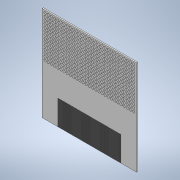
# Autodesk Inventor part: CeramicPCB_Coarse
Saved by Autodesk Inventor 2021 (Build 250183000, 183)
## iProperties
Created: 2021-11-05
Part Number: CeramicPCB_Coarse
Material: Generic
Document SubType Name: Sheet Metal
Designer: Unit-005
Density: 1 g/cm^3
Sheet Metal Rule: Default
Appearance: Default
Author: Unit-005
Autodesk Inventor part; units mm, degrees
ref_plane "YZ Plane" through (0, 0, 0) normal (1, 0, 0) x (0, 1, 0)
ref_plane "XZ Plane" through (0, 0, 0) normal (0, 1, 0) x (-1, 0, 0)
ref_plane "XY Plane" through (0, 0, 0) normal (0, 0, 1) x (1, 0, 0)
sketch "Sketch1" plane through (0, 0, 0) normal (0, 0, 1) x (1, 0, 0)
  line L0 (-38, 38) -> (38, 38)
  line L1 (38, 38) -> (38, -38)
  line L2 (38, -38) -> (-38, -38)
  line L3 (-38, -38) -> (-38, 38)
  line L4 (-38, 38) -> (38, -38) construction
  line L5 (38, 38) -> (-38, -38) construction
  point P0 (0, 0)
  dimension "d0" = 76
  dimension "d1" = 76
  constraints: 12 end point, 2 midpoint, 2 parallel, 1 horizontal, 1 perpendicular
  measures "d0" distance of L1.end L2.end
  measures "d1" distance of L0.end L1.end
extrude "Extrusion1" add sketch "Sketch1" along normal blind 1
sketch "Sketch2" plane through (0, 0, 1) normal (0, 0, 1) x (1, 0, 0)
  line L0 (-38, -38) -> (38, -38) projected
  line L1 (38, -38) -> (38, 38) projected
  line L2 (38, 38) -> (-38, 38) projected
  line L3 (-38, 38) -> (-38, -38) projected
  line L4 (-53.2, 0) -> (53.2, 0) projected
  line L5 (0, -53.2) -> (0, 53.2) projected
  line L6 (-0.15, -18) -> (0.15, -18)
  line L7 (0.15, -18) -> (0.15, -38)
  line L8 (0.15, -38) -> (-0.15, -38)
  line L9 (-0.15, -38) -> (-0.15, -18)
  line L10 (-0.15, -18) -> (0.15, -38) construction
  line L11 (0.15, -18) -> (-0.15, -38) construction
  line L12 (-38, -38) -> (38, -38) projected
  point P0 (0, 0)
  point P1 (0, -28)
  dimension "d4" = 0.3
  dimension "d5" = 20
  constraints: 12 end point, 2 midpoint, 2 parallel, 1 collinear, 1 horizontal, 1 perpendicular, 1 point on line
  measures "d4" distance of L7.end L8.end
  measures "d5" distance of L6.end L7.end
extrude "Extrusion2" add sketch "Sketch2" along normal blind 0.035 contours L9 L6 L5 L0 | L5 L6 L7 L0
pattern_linear "Rectangular Pattern1" count 85 spacing 0.6 along (1, 0, 0) of "Extrusion2" first direction both ways yes
sketch "Sketch3" plane through (0, 0, 1) normal (0, 0, 1) x (1, 0, 0)
  line L0 (0.15, -38) -> (0.45, -38) projected
  line L1 (38, -38) -> (38, 38) projected
  line L2 (38, 38) -> (-38, 38) projected
  line L3 (-38, 38) -> (-38, -38) projected
  line L4 (-38, -38) -> (-25.35, -38) projected
  line L5 (-53.2, 0) -> (53.2, 0) projected
  line L6 (0, -53.2) -> (0, 53.2) projected
  line L7 (33, -38) -> (33, 2) construction
  line L8 (-25.05, -38) -> (-24.75, -38) projected
  line L9 (-24.45, -38) -> (-24.15, -38) projected
  line L10 (-22.35, -38) -> (-22.35, -18) projected
  line L11 (-22.35, -18) -> (-22.05, -18) projected
  line L12 (-22.05, -18) -> (-22.05, -38) projected
  line L13 (-22.05, -38) -> (-21.75, -38) projected
  line L14 (-21.75, -38) -> (-21.75, -18) projected
  line L15 (-21.75, -18) -> (-21.45, -18) projected
  line L16 (-21.45, -18) -> (-21.45, -38) projected
  line L17 (-21.45, -38) -> (-21.15, -38) projected
  line L18 (-21.15, -38) -> (-21.15, -18) projected
  line L19 (-21.15, -18) -> (-20.85, -18) projected
  line L20 (-20.85, -18) -> (-20.85, -38) projected
  line L21 (-20.85, -38) -> (-20.55, -38) projected
  line L22 (-20.55, -38) -> (-20.55, -18) projected
  line L23 (-20.55, -18) -> (-20.25, -18) projected
  line L24 (-20.25, -18) -> (-20.25, -38) projected
  line L25 (-20.25, -38) -> (-19.95, -38) projected
  line L26 (-19.95, -38) -> (-19.95, -18) projected
  line L27 (-19.95, -18) -> (-19.65, -18) projected
  line L28 (-19.65, -18) -> (-19.65, -38) projected
  line L29 (-19.65, -38) -> (-19.35, -38) projected
  line L30 (-19.35, -38) -> (-19.35, -18) projected
  line L31 (-19.35, -18) -> (-19.05, -18) projected
  line L32 (-19.05, -18) -> (-19.05, -38) projected
  line L33 (-19.05, -38) -> (-18.75, -38) projected
  line L34 (-18.75, -38) -> (-18.75, -18) projected
  line L35 (-18.75, -18) -> (-18.45, -18) projected
  line L36 (-18.45, -18) -> (-18.45, -38) projected
  line L37 (-18.45, -38) -> (-18.15, -38) projected
  line L38 (-18.15, -38) -> (-18.15, -18) projected
  line L39 (-18.15, -18) -> (-17.85, -18) projected
  line L40 (-17.85, -18) -> (-17.85, -38) projected
  line L41 (-17.85, -38) -> (-17.55, -38) projected
  line L42 (-17.55, -38) -> (-17.55, -18) projected
  line L43 (-17.55, -18) -> (-17.25, -18) projected
  line L44 (-17.25, -18) -> (-17.25, -38) projected
  line L45 (-17.25, -38) -> (-16.95, -38) projected
  line L46 (-16.95, -38) -> (-16.95, -18) projected
  line L47 (-16.95, -18) -> (-16.65, -18) projected
  line L48 (-16.65, -18) -> (-16.65, -38) projected
  line L49 (-16.65, -38) -> (-16.35, -38) projected
  line L50 (-16.35, -38) -> (-16.35, -18) projected
  line L51 (-16.35, -18) -> (-16.05, -18) projected
  line L52 (-16.05, -18) -> (-16.05, -38) projected
  line L53 (-16.05, -38) -> (-15.75, -38) projected
  line L54 (-15.75, -38) -> (-15.75, -18) projected
  line L55 (-15.75, -18) -> (-15.45, -18) projected
  line L56 (-15.45, -18) -> (-15.45, -38) projected
  line L57 (-15.15, -38) -> (-15.15, -18) projected
  line L58 (-15.15, -18) -> (-14.85, -18) projected
  line L59 (-14.85, -18) -> (-14.85, -38) projected
  line L60 (-14.85, -38) -> (-14.55, -38) projected
  line L61 (-14.55, -38) -> (-14.55, -18) projected
  line L62 (-14.55, -18) -> (-14.25, -18) projected
  line L63 (-14.25, -18) -> (-14.25, -38) projected
  line L64 (-14.25, -38) -> (-13.95, -38) projected
  line L65 (-13.95, -38) -> (-13.95, -18) projected
  line L66 (-13.95, -18) -> (-13.65, -18) projected
  line L67 (-13.65, -18) -> (-13.65, -38) projected
  line L68 (-13.65, -38) -> (-13.35, -38) projected
  line L69 (-13.35, -38) -> (-13.35, -18) projected
  line L70 (-13.35, -18) -> (-13.05, -18) projected
  line L71 (-13.05, -18) -> (-13.05, -38) projected
  line L72 (-13.05, -38) -> (-12.75, -38) projected
  line L73 (-12.75, -38) -> (-12.75, -18) projected
  line L74 (-12.75, -18) -> (-12.45, -18) projected
  line L75 (-12.45, -18) -> (-12.45, -38) projected
  line L76 (-12.45, -38) -> (-12.15, -38) projected
  line L77 (-12.15, -38) -> (-12.15, -18) projected
  line L78 (-12.15, -18) -> (-11.85, -18) projected
  line L79 (-11.85, -18) -> (-11.85, -38) projected
  line L80 (-11.85, -38) -> (-11.55, -38) projected
  line L81 (-11.55, -38) -> (-11.55, -18) projected
  line L82 (-11.55, -18) -> (-11.25, -18) projected
  line L83 (-11.25, -18) -> (-11.25, -38) projected
  line L84 (-11.25, -38) -> (-10.95, -38) projected
  line L85 (-10.95, -38) -> (-10.95, -18) projected
  line L86 (-10.95, -18) -> (-10.65, -18) projected
  line L87 (-10.65, -18) -> (-10.65, -38) projected
  line L88 (-10.65, -38) -> (-10.35, -38) projected
  line L89 (-10.35, -38) -> (-10.35, -18) projected
  line L90 (-10.35, -18) -> (-10.05, -18) projected
  line L91 (-10.05, -18) -> (-10.05, -38) projected
  line L92 (-10.05, -38) -> (-9.75, -38) projected
  line L93 (-9.75, -38) -> (-9.75, -18) projected
  line L94 (-9.75, -18) -> (-9.45, -18) projected
  line L95 (-9.45, -18) -> (-9.45, -38) projected
  line L96 (-9.45, -38) -> (-9.15, -38) projected
  line L97 (-9.15, -38) -> (-9.15, -18) projected
  line L98 (-9.15, -18) -> (-8.85, -18) projected
  line L99 (-8.85, -18) -> (-8.85, -38) projected
  line L100 (-8.85, -38) -> (-8.55, -38) projected
  line L101 (-8.55, -38) -> (-8.55, -18) projected
  line L102 (-8.55, -18) -> (-8.25, -18) projected
  line L103 (-8.25, -18) -> (-8.25, -38) projected
  line L104 (-8.25, -38) -> (-7.95, -38) projected
  line L105 (-7.95, -38) -> (-7.95, -18) projected
  line L106 (-7.95, -18) -> (-7.65, -18) projected
  line L107 (-7.65, -18) -> (-7.65, -38) projected
  line L108 (-7.65, -38) -> (-7.35, -38) projected
  line L109 (-7.35, -38) -> (-7.35, -18) projected
  line L110 (-7.35, -18) -> (-7.05, -18) projected
  line L111 (-7.05, -18) -> (-7.05, -38) projected
  line L112 (-7.05, -38) -> (-6.75, -38) projected
  line L113 (-6.75, -38) -> (-6.75, -18) projected
  line L114 (-6.75, -18) -> (-6.45, -18) projected
  line L115 (-6.45, -18) -> (-6.45, -38) projected
  line L116 (-6.45, -38) -> (-6.15, -38) projected
  line L117 (-6.15, -38) -> (-6.15, -18) projected
  line L118 (-6.15, -18) -> (-5.85, -18) projected
  line L119 (-5.85, -18) -> (-5.85, -38) projected
  line L120 (-5.85, -38) -> (-5.55, -38) projected
  line L121 (-5.55, -38) -> (-5.55, -18) projected
  line L122 (-5.55, -18) -> (-5.25, -18) projected
  line L123 (-5.25, -18) -> (-5.25, -38) projected
  line L124 (-5.25, -38) -> (-4.95, -38) projected
  line L125 (-4.95, -38) -> (-4.95, -18) projected
  line L126 (-4.95, -18) -> (-4.65, -18) projected
  line L127 (-4.65, -18) -> (-4.65, -38) projected
  line L128 (-4.65, -38) -> (-4.35, -38) projected
  line L129 (-4.35, -38) -> (-4.35, -18) projected
  line L130 (-4.35, -18) -> (-4.05, -18) projected
  line L131 (-4.05, -18) -> (-4.05, -38) projected
  line L132 (-4.05, -38) -> (-3.75, -38) projected
  line L133 (-3.75, -38) -> (-3.75, -18) projected
  line L134 (-3.75, -18) -> (-3.45, -18) projected
  line L135 (-3.45, -18) -> (-3.45, -38) projected
  line L136 (-3.45, -38) -> (-3.15, -38) projected
  line L137 (-3.15, -38) -> (-3.15, -18) projected
  line L138 (-3.15, -18) -> (-2.85, -18) projected
  line L139 (-2.85, -18) -> (-2.85, -38) projected
  line L140 (-2.85, -38) -> (-2.55, -38) projected
  line L141 (-2.55, -38) -> (-2.55, -18) projected
  line L142 (-2.55, -18) -> (-2.25, -18) projected
  line L143 (-2.25, -18) -> (-2.25, -38) projected
  line L144 (-2.25, -38) -> (-1.95, -38) projected
  line L145 (-1.95, -38) -> (-1.95, -18) projected
  line L146 (-1.95, -18) -> (-1.65, -18) projected
  line L147 (-1.65, -18) -> (-1.65, -38) projected
  line L148 (-1.65, -38) -> (-1.35, -38) projected
  line L149 (-1.35, -38) -> (-1.35, -18) projected
  line L150 (-1.35, -18) -> (-1.05, -18) projected
  line L151 (-1.05, -18) -> (-1.05, -38) projected
  line L152 (-1.05, -38) -> (-0.75, -38) projected
  line L153 (-0.75, -38) -> (-0.75, -18) projected
  line L154 (-0.75, -18) -> (-0.45, -18) projected
  line L155 (-0.45, -18) -> (-0.45, -38) projected
  line L156 (-0.45, -38) -> (-0.15, -38) projected
  line L157 (-0.15, -38) -> (-0.15, -18) projected
  line L158 (-0.15, -18) -> (0.15, -18) projected
  line L159 (0.15, -18) -> (0.15, -38) projected
  line L160 (0.45, -38) -> (0.45, -18) projected
  line L161 (0.45, -18) -> (0.75, -18) projected
  line L162 (0.75, -18) -> (0.75, -38) projected
  line L163 (0.75, -38) -> (1.05, -38) projected
  line L164 (1.05, -38) -> (1.05, -18) projected
  line L165 (1.05, -18) -> (1.35, -18) projected
  line L166 (1.35, -18) -> (1.35, -38) projected
  line L167 (1.35, -38) -> (1.65, -38) projected
  line L168 (1.65, -38) -> (1.65, -18) projected
  line L169 (1.65, -18) -> (1.95, -18) projected
  line L170 (1.95, -18) -> (1.95, -38) projected
  line L171 (1.95, -38) -> (2.25, -38) projected
  line L172 (2.25, -38) -> (2.25, -18) projected
  line L173 (2.25, -18) -> (2.55, -18) projected
  line L174 (2.55, -18) -> (2.55, -38) projected
  line L175 (2.55, -38) -> (2.85, -38) projected
  line L176 (2.85, -38) -> (2.85, -18) projected
  line L177 (2.85, -18) -> (3.15, -18) projected
  line L178 (3.15, -18) -> (3.15, -38) projected
  line L179 (3.15, -38) -> (3.45, -38) projected
  line L180 (3.45, -38) -> (3.45, -18) projected
  line L181 (3.45, -18) -> (3.75, -18) projected
  line L182 (3.75, -18) -> (3.75, -38) projected
  line L183 (3.75, -38) -> (4.05, -38) projected
  line L184 (4.05, -38) -> (4.05, -18) projected
  line L185 (4.05, -18) -> (4.35, -18) projected
  line L186 (4.35, -18) -> (4.35, -38) projected
  line L187 (4.35, -38) -> (4.65, -38) projected
  line L188 (4.65, -38) -> (4.65, -18) projected
  line L189 (4.65, -18) -> (4.95, -18) projected
  line L190 (4.95, -18) -> (4.95, -38) projected
  line L191 (4.95, -38) -> (5.25, -38) projected
  line L192 (5.25, -38) -> (5.25, -18) projected
  line L193 (5.25, -18) -> (5.55, -18) projected
  line L194 (5.55, -18) -> (5.55, -38) projected
  line L195 (5.55, -38) -> (5.85, -38) projected
  line L196 (5.85, -38) -> (5.85, -18) projected
  line L197 (5.85, -18) -> (6.15, -18) projected
  line L198 (6.15, -18) -> (6.15, -38) projected
  line L199 (6.15, -38) -> (6.45, -38) projected
  line L200 (6.45, -38) -> (6.45, -18) projected
  line L201 (6.45, -18) -> (6.75, -18) projected
  line L202 (6.75, -18) -> (6.75, -38) projected
  line L203 (6.75, -38) -> (7.05, -38) projected
  line L204 (7.05, -38) -> (7.05, -18) projected
  line L205 (7.05, -18) -> (7.35, -18) projected
  line L206 (7.35, -18) -> (7.35, -38) projected
  line L207 (7.35, -38) -> (7.65, -38) projected
  line L208 (7.65, -38) -> (7.65, -18) projected
  line L209 (7.65, -18) -> (7.95, -18) projected
  line L210 (7.95, -18) -> (7.95, -38) projected
  line L211 (7.95, -38) -> (8.25, -38) projected
  line L212 (8.25, -38) -> (8.25, -18) projected
  line L213 (8.25, -18) -> (8.55, -18) projected
  line L214 (8.55, -18) -> (8.55, -38) projected
  line L215 (8.55, -38) -> (8.85, -38) projected
  line L216 (8.85, -38) -> (8.85, -18) projected
  line L217 (8.85, -18) -> (9.15, -18) projected
  line L218 (9.15, -18) -> (9.15, -38) projected
  line L219 (9.15, -38) -> (9.45, -38) projected
  line L220 (9.45, -38) -> (9.45, -18) projected
  line L221 (9.45, -18) -> (9.75, -18) projected
  line L222 (9.75, -18) -> (9.75, -38) projected
  line L223 (9.75, -38) -> (10.05, -38) projected
  line L224 (10.05, -38) -> (10.05, -18) projected
  line L225 (10.05, -18) -> (10.35, -18) projected
  line L226 (10.35, -18) -> (10.35, -38) projected
  line L227 (10.35, -38) -> (10.65, -38) projected
  line L228 (10.65, -38) -> (10.65, -18) projected
  line L229 (10.65, -18) -> (10.95, -18) projected
  line L230 (10.95, -18) -> (10.95, -38) projected
  line L231 (10.95, -38) -> (11.25, -38) projected
  line L232 (11.25, -38) -> (11.25, -18) projected
  line L233 (11.25, -18) -> (11.55, -18) projected
  line L234 (11.55, -18) -> (11.55, -38) projected
  line L235 (11.55, -38) -> (11.85, -38) projected
  line L236 (11.85, -38) -> (11.85, -18) projected
  line L237 (11.85, -18) -> (12.15, -18) projected
  line L238 (12.15, -18) -> (12.15, -38) projected
  line L239 (12.15, -38) -> (12.45, -38) projected
  line L240 (12.45, -38) -> (12.45, -18) projected
  line L241 (12.45, -18) -> (12.75, -18) projected
  line L242 (12.75, -18) -> (12.75, -38) projected
  line L243 (12.75, -38) -> (13.05, -38) projected
  line L244 (13.05, -38) -> (13.05, -18) projected
  line L245 (13.05, -18) -> (13.35, -18) projected
  line L246 (13.35, -18) -> (13.35, -38) projected
  line L247 (13.35, -38) -> (13.65, -38) projected
  line L248 (13.65, -38) -> (13.65, -18) projected
  line L249 (13.65, -18) -> (13.95, -18) projected
  line L250 (13.95, -18) -> (13.95, -38) projected
  line L251 (13.95, -38) -> (14.25, -38) projected
  line L252 (14.25, -38) -> (14.25, -18) projected
  line L253 (14.25, -18) -> (14.55, -18) projected
  line L254 (14.55, -18) -> (14.55, -38) projected
  line L255 (14.55, -38) -> (14.85, -38) projected
  line L256 (14.85, -38) -> (14.85, -18) projected
  line L257 (14.85, -18) -> (15.15, -18) projected
  line L258 (15.15, -18) -> (15.15, -38) projected
  line L259 (15.15, -38) -> (15.45, -38) projected
  line L260 (15.45, -38) -> (15.45, -18) projected
  line L261 (15.45, -18) -> (15.75, -18) projected
  line L262 (15.75, -18) -> (15.75, -38) projected
  line L263 (15.75, -38) -> (16.05, -38) projected
  line L264 (16.05, -38) -> (16.05, -18) projected
  line L265 (16.05, -18) -> (16.35, -18) projected
  line L266 (16.35, -18) -> (16.35, -38) projected
  line L267 (16.35, -38) -> (16.65, -38) projected
  line L268 (16.65, -38) -> (16.65, -18) projected
  line L269 (16.65, -18) -> (16.95, -18) projected
  line L270 (16.95, -18) -> (16.95, -38) projected
  line L271 (16.95, -38) -> (17.25, -38) projected
  line L272 (17.25, -38) -> (17.25, -18) projected
  line L273 (17.25, -18) -> (17.55, -18) projected
  line L274 (17.55, -18) -> (17.55, -38) projected
  line L275 (17.55, -38) -> (17.85, -38) projected
  line L276 (17.85, -38) -> (17.85, -18) projected
  line L277 (17.85, -18) -> (18.15, -18) projected
  line L278 (18.15, -18) -> (18.15, -38) projected
  line L279 (18.15, -38) -> (18.45, -38) projected
  line L280 (18.45, -38) -> (18.45, -18) projected
  line L281 (18.45, -18) -> (18.75, -18) projected
  line L282 (18.75, -18) -> (18.75, -38) projected
  line L283 (18.75, -38) -> (19.05, -38) projected
  line L284 (19.05, -38) -> (19.05, -18) projected
  line L285 (19.05, -18) -> (19.35, -18) projected
  line L286 (19.35, -18) -> (19.35, -38) projected
  line L287 (19.35, -38) -> (19.65, -38) projected
  line L288 (19.65, -38) -> (19.65, -18) projected
  line L289 (19.65, -18) -> (19.95, -18) projected
  line L290 (19.95, -18) -> (19.95, -38) projected
  line L291 (19.95, -38) -> (20.25, -38) projected
  line L292 (20.25, -38) -> (20.25, -18) projected
  line L293 (20.25, -18) -> (20.55, -18) projected
  line L294 (20.55, -18) -> (20.55, -38) projected
  line L295 (20.55, -38) -> (20.85, -38) projected
  line L296 (20.85, -38) -> (20.85, -18) projected
  line L297 (20.85, -18) -> (21.15, -18) projected
  line L298 (21.15, -18) -> (21.15, -38) projected
  line L299 (21.15, -38) -> (21.45, -38) projected
  line L300 (21.45, -38) -> (21.45, -18) projected
  line L301 (21.45, -18) -> (21.75, -18) projected
  line L302 (21.75, -18) -> (21.75, -38) projected
  line L303 (21.75, -38) -> (22.05, -38) projected
  line L304 (22.05, -38) -> (22.05, -18) projected
  line L305 (22.05, -18) -> (22.35, -18) projected
  line L306 (22.35, -18) -> (22.35, -38) projected
  line L307 (25.35, -18) -> (25.35, -38) projected
  line L308 (25.35, -38) -> (38, -38) projected
  line L309 (-25.35, -38) -> (-25.35, -18) projected
  line L310 (-25.35, -18) -> (-25.05, -18) projected
  line L311 (-25.05, -18) -> (-25.05, -38) projected
  line L312 (-24.75, -38) -> (-24.75, -18) projected
  line L313 (-24.75, -18) -> (-24.45, -18) projected
  line L314 (-24.45, -18) -> (-24.45, -38) projected
  line L315 (-24.15, -38) -> (-24.15, -18) projected
  line L316 (-24.15, -18) -> (-23.85, -18) projected
  line L317 (-23.85, -18) -> (-23.85, -38) projected
  line L318 (-23.85, -38) -> (-23.55, -38) projected
  line L319 (-23.55, -38) -> (-23.55, -18) projected
  line L320 (-23.55, -18) -> (-23.25, -18) projected
  line L321 (-23.25, -18) -> (-23.25, -38) projected
  line L322 (-23.25, -38) -> (-22.95, -38) projected
  line L323 (-22.95, -38) -> (-22.95, -18) projected
  line L324 (-22.95, -18) -> (-22.65, -18) projected
  line L325 (-22.65, -18) -> (-22.65, -38) projected
  line L326 (-22.65, -38) -> (-22.35, -38) projected
  line L327 (-15.45, -38) -> (-15.15, -38) projected
  line L328 (22.35, -38) -> (22.65, -38) projected
  line L329 (22.65, -38) -> (22.65, -18) projected
  line L330 (22.65, -18) -> (22.95, -18) projected
  line L331 (22.95, -18) -> (22.95, -38) projected
  line L332 (22.95, -38) -> (23.25, -38) projected
  line L333 (23.25, -38) -> (23.25, -18) projected
  line L334 (23.25, -18) -> (23.55, -18) projected
  line L335 (23.55, -18) -> (23.55, -38) projected
  line L336 (23.55, -38) -> (23.85, -38) projected
  line L337 (23.85, -38) -> (23.85, -18) projected
  line L338 (23.85, -18) -> (24.15, -18) projected
  line L339 (24.15, -18) -> (24.15, -38) projected
  line L340 (24.15, -38) -> (24.45, -38) projected
  line L341 (24.45, -38) -> (24.45, -18) projected
  line L342 (24.45, -18) -> (24.75, -18) projected
  line L343 (24.75, -18) -> (24.75, -38) projected
  line L344 (24.75, -38) -> (25.05, -38) projected
  line L345 (25.05, -38) -> (25.05, -18) projected
  line L346 (25.05, -18) -> (25.35, -18) projected
  circle A0 centre (0, 36) radius 1
  point P0 (0, 0)
  dimension "d11" = 40
  dimension "d12" = 5
  dimension "d13" = 2
  dimension "d18" = 2
  constraints: 2 end point, 2 point on line, 1 centre point, 1 perpendicular
  measures "d11" distance of L7.start L7.end
  measures "d12" distance between parallel lines of L1 L7
  measures "d13" diameter of A0
  measures "d18" distance from line of L2 A0.centre
extrude "Extrusion3" add sketch "Sketch3" along normal blind 0.035 contours A0 L6 | L6 A0
pattern_linear "Rectangular Pattern2" count 29 spacing 2.54 along (1, 0, 0) count 14 spacing 2.54 along (0, -1, 0) of "Extrusion3" first direction both ways yes
equation "\"BendRadius\" = Thickness"
equation "\"BendReliefWidth\" = Thickness"
equation "\"BendReliefDepth\" = 0.5 * Thickness"
equation "\"CornerReliefSize\" = 4 * Thickness"
equation "\"MinimumRemnant\" = 2 * Thickness"
equation "\"TransitionRadius\" = BendRadius"
equation "\"JacobiRadiusSize\" = BendRadius"
equation "\"GapSize\" = Thickness"
equation "\"Thickness\" = 3.048"
body "Solid1"
